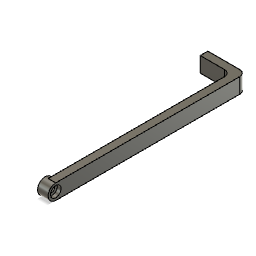
toolbox-handle-holder (Autodesk Fusion 360 design; units mm, degrees)
Autodesk Fusion 360 part; units mm, degrees
sketch "Sketch1" plane through (0, 0, 0) normal (0, 1, 0) x (1, 0, 0)
  line L0 (0, 0) -> (25, 0) construction
  line L1 (25, 0) -> (25, 130) construction
  line L2 (25, 130) -> (0, 130) construction
  line L3 (0, 130) -> (0, 0) construction
  line L4 (25, 0) -> (20, 0)
  line L5 (0, 130) -> (0, 125)
  line L6 (20, 121) -> (20, 0)
  line L7 (25, 0) -> (25, 126)
  line L8 (0, 130) -> (21, 130)
  line L9 (16, 125) -> (0, 125)
  arc A0 (20, 121) -> (16, 125) centre (16, 121) ccw
  arc A1 (25, 126) -> (21, 130) centre (21, 126) ccw
  dimension "d1" = 25
  dimension "d2" = 130
  dimension "d3" = 5
  dimension "d4" = 4
  dimension "d5" = 4
  dimension "d18" = 5
  constraint horizontal L0
  constraint vertical L1
  constraint horizontal L2
  constraint vertical L3
  constraint coincident L0.start L3.end
  constraint perpendicular L1 L4
  constraint coincident L3 L5.end
  constraint perpendicular L0 L6
  constraint perpendicular L3 L9
  constraint tangent L9 A0
  constraint tangent L6 A0
  constraint coincident L1.end L8
  constraint coincident L1.end L7
  constraint tangent L8 A1
  constraint tangent L7 A1
  measures "d1" distance of L0.start L0.end
  measures "d2" distance of L0.start L2.end
  measures "d3" distance of L0.end L4.end
  measures "d4" radius of A0
  measures "d5" radius of A1
  measures "d18" distance of L8 L9
extrude "Extrude1" add sketch "Sketch1" along normal blind 10
fillet "Fillet1" radius 5 2 edges at (22.5, 10, 0) (22.5, 0, 0)
sketch "Sketch2" plane through (25, 0, 0) normal (1, 0, 0) x (0, 0, -1)
  arc A0 (5, 10) -> (5, 0) centre (5, 5) ccw
  line L0 (5, 0) -> (126, 0)
  line L1 (126, 0) -> (126, 10)
  line L2 (126, 10) -> (5, 10)
  line L3 (0, 5) -> (5, 5) construction
  circle A1 centre (5, 5) radius 1.75
  circle A2 centre (5, 5) radius 3.5
  dimension "d9" = 5
  dimension "d10" = 3.5
  dimension "d11" = 7
  constraint midpoint A0 L3.start
  constraint horizontal L3
  constraint coincident A0.centre L3.end
  constraint concentric A1 A2
  measures "d9" distance of L3.start A0.centre
  measures "d10" diameter of A1
  measures "d11" diameter of A2
extrude "Extrude2" cut sketch "Sketch2" against normal up to surface (5 mm away) contours A1
extrude "Extrude3" cut sketch "Sketch2" against normal blind 2.5 contours A2
sketch "Sketch3" plane through (20, 0, 0) normal (-1, 0, 0) x (0, 0, 1)
  circle A0 centre (-5, 5) radius 1.75
  arc A1 (-5, 0) -> (-5, 10) centre (-5, 5) ccw
  line L0 (-5, 10) -> (-121, 10)
  line L1 (-121, 10) -> (-121, 0)
  line L2 (-121, 0) -> (-5, 0)
  circle A2 centre (-5, 5) radius 5
  constraint concentric A0 A2
extrude "Extrude4" add sketch "Sketch3" along normal blind 2 contours A1 A2
